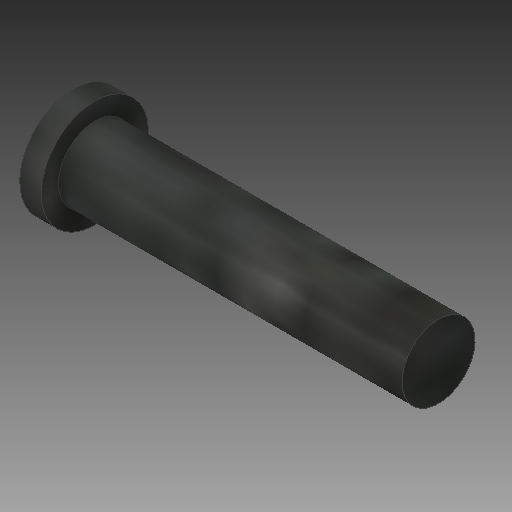
# Autodesk Inventor part: M2_L10
Saved by Autodesk Inventor 2018 (Build 220112000, 112)
## iProperties
Part Number: M2_L10
Material: 鋼
Document SubType Name: Modeling
Designer: sktom
Density: 7.85 g/cm^3
Appearance: プレート
Author: sktom
Autodesk Inventor part; units mm, degrees
ref_plane "YZ Plane" through (0, 0, 0) normal (1, 0, 0) x (0, 1, 0)
ref_plane "XZ Plane" through (0, 0, 0) normal (0, 1, 0) x (-1, 0, 0)
ref_plane "XY Plane" through (0, 0, 0) normal (0, 0, 1) x (1, 0, 0)
sketch "スケッチ1" plane through (0, 0, 0) normal (0, 0, 1) x (1, 0, 0)
  line L0 (0, 0) -> (0, 1.25)
  line L1 (0, 1.25) -> (0.5, 1.25)
  line L2 (0.5, 1.25) -> (0.5, 0.85)
  line L3 (0.5, 0.85) -> (8.5, 0.85)
  line L4 (8.5, 0.85) -> (8.5, 0)
  line L5 (8.5, 0) -> (0, 0)
  dimension "d0" = 0.5
  dimension "d1" = 8
  dimension "d2" = 1.25
  dimension "d3" = 0.85
  constraints: 12 end point, 5 perpendicular, 1 vertical
  measures "d0" distance of L0.end L1.end
  measures "d1" distance of L2.end L3.end
  measures "d2" distance between parallel lines of L5 L1
  measures "d3" distance between parallel lines of L5 L3
revolve "回転1" add sketch "スケッチ1" angle 360 about axis through (8.5, 0, 0) along (-1, 0, 0)
